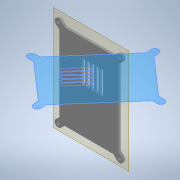
# Autodesk Inventor part: CoverWFan
Saved by Autodesk Inventor 2021 (Build 250183000, 183)
## iProperties
Created: 2021-07-24
Part Number: CoverWFan
Material: ABS Plastic
Document SubType Name: Modeling
Designer: cmzgt
Density: 1.06 g/cm^3
Appearance: Smooth - White
Author: cmzgt
Autodesk Inventor part; units mm, degrees
ref_plane "YZ Plane" through (0, 0, 0) normal (1, 0, 0) x (0, 1, 0)
ref_plane "XZ Plane" through (0, 0, 0) normal (0, 1, 0) x (-1, 0, 0)
ref_plane "XY Plane" through (0, 0, 0) normal (0, 0, 1) x (1, 0, 0)
ref_plane "Work Plane1" through (0, 0, 0) normal (0, 0, 1) x (1, 0, 0)
sketch "Sketch1" plane through (0, 0, 0) normal (0, 0, 1) x (1, 0, 0)
  line L0 (162.668, -44.5954) -> (162.668, 41.2818) projected
  line L1 (166.8059, 44.8966) -> (162.668, 41.2818) projected
  arc A0 (166.8059, 44.8966) -> (161.5426, 50.9214) centre (164.1742, 47.909) ccw projected
  circle A1 centre (164.1742, 47.909) radius 1.375 projected
  line L2 (158.5302, 48.2898) -> (161.5426, 50.9214) projected
  arc A2 (158.5302, 48.2898) -> (157.3844, 46.5932) centre (161.1618, 45.2774) ccw projected
  line L3 (157.3844, 46.5932) -> (101.3516, 46.5932) projected
  arc A3 (101.3516, 46.5932) -> (100.2059, 48.2898) centre (97.5742, 45.2774) ccw projected
  line L4 (97.1935, 50.9214) -> (100.2059, 48.2898) projected
  arc A4 (97.1935, 50.9214) -> (91.9302, 44.8966) centre (94.5618, 47.909) ccw projected
  circle A5 centre (94.5618, 47.909) radius 1.375 projected
  line L5 (96.068, 41.2818) -> (91.9302, 44.8966) projected
  line L6 (96.068, 41.2818) -> (96.068, -44.5954) projected
  line L7 (91.9302, -48.2102) -> (96.068, -44.5954) projected
  arc A6 (91.9302, -48.2102) -> (97.1935, -54.235) centre (94.5618, -51.2226) ccw projected
  line L8 (100.2059, -51.6034) -> (97.1935, -54.235) projected
  arc A7 (100.2059, -51.6034) -> (101.3516, -49.9068) centre (97.5742, -48.591) ccw projected
  circle A8 centre (94.5618, -51.2226) radius 1.375 projected
  line L9 (101.3516, -49.9068) -> (157.3844, -49.9068) projected
  line L10 (161.5426, -54.235) -> (158.5302, -51.6034) projected
  arc A9 (157.3844, -49.9068) -> (158.5302, -51.6034) centre (161.1618, -48.591) ccw projected
  arc A10 (161.5426, -54.235) -> (166.8059, -48.2102) centre (164.1742, -51.2226) ccw projected
  line L11 (162.668, -44.5954) -> (166.8059, -48.2102) projected
  circle A11 centre (164.1742, -51.2226) radius 1.375 projected
  line L12 (102.868, 42.7932) -> (155.868, 42.7932) projected
  arc A12 (158.868, 39.7932) -> (155.868, 42.7932) centre (155.868, 39.7932) ccw projected
  line L13 (158.868, 39.7932) -> (158.868, -43.1068) projected
  arc A13 (155.868, -46.1068) -> (158.868, -43.1068) centre (155.868, -43.1068) ccw projected
  line L14 (155.868, -46.1068) -> (102.868, -46.1068) projected
  arc A14 (99.868, -43.1068) -> (102.868, -46.1068) centre (102.868, -43.1068) ccw projected
  line L15 (99.868, -43.1068) -> (99.868, 39.7932) projected
  arc A15 (102.868, 42.7932) -> (99.868, 39.7932) centre (102.868, 39.7932) ccw projected
  point P0 (0, 0)
  point P1 (-32.2078, 42.9557)
  point P2 (-31.0209, 50.8588)
  point P3 (-31.2556, 42.9706)
  point P4 (90.7091, 46.8336)
  point P5 (90.8754, -49.6701)
  point P6 (94.8543, -45.6557)
  point P7 (38.6589, -48.4904)
  point P8 (35.6268, 48.0781)
extrude "Extrusion1" add sketch "Sketch1" along normal blind 2.5 contours L11 A10 L10 A9 L9 A7 L8 A6 L7 L6 L5 A4 L4 A3 L3 A2 L2 A0 L1 L0 | A1 | A5 | A8 | A11 | L12 A12 L13 A13 L14 A14 L15 A15
sketch "Sketch2" plane through (0, 0, 2.5) normal (0, 0, 1) x (1, 0, 0)
  line L0 (140.3574, 20.4135) -> (126.2672, 20.4135) construction
  line L1 (126.2672, 20.4135) -> (126.2672, 6.3233) construction
  line L2 (126.2672, 6.3233) -> (140.3574, 6.3233) construction
  line L3 (140.3574, 6.3233) -> (140.3574, 20.4135) construction
  line L4 (133.3123, 25.0032) -> (133.3123, 2.1432) construction
  line L5 (131.4073, 25.0032) -> (131.4073, 2.1432)
  line L6 (135.2173, 2.1432) -> (135.2173, 25.0032)
  arc A0 (135.2173, 25.0032) -> (131.4073, 25.0032) centre (133.3123, 25.0032) ccw
  arc A1 (131.4073, 2.1432) -> (135.2173, 2.1432) centre (133.3123, 2.1432) ccw
  line L7 (162.668, -44.5954) -> (162.668, 41.2818) projected
  line L8 (157.3844, 46.5932) -> (101.3516, 46.5932) projected
  line L9 (140.2973, 2.1432) -> (140.2973, 25.0032)
  arc A2 (140.2973, 25.0032) -> (136.4873, 25.0032) centre (138.3923, 25.0032) ccw
  line L10 (136.4873, 25.0032) -> (136.4873, 2.1432)
  arc A3 (136.4873, 2.1432) -> (140.2973, 2.1432) centre (138.3923, 2.1432) ccw
  line L11 (145.3773, 2.1432) -> (145.3773, 25.0032)
  arc A4 (145.3773, 25.0032) -> (141.5673, 25.0032) centre (143.4723, 25.0032) ccw
  line L12 (141.5673, 25.0032) -> (141.5673, 2.1432)
  arc A5 (141.5673, 2.1432) -> (145.3773, 2.1432) centre (143.4723, 2.1432) ccw
  arc A6 (130.1373, 25.0032) -> (126.3273, 25.0032) centre (128.2323, 25.0032) ccw
  line L13 (130.1373, 2.1432) -> (130.1373, 25.0032)
  line L14 (126.3273, 25.0032) -> (126.3273, 2.1432)
  arc A7 (126.3273, 2.1432) -> (130.1373, 2.1432) centre (128.2323, 2.1432) ccw
  arc A8 (125.0573, 25.0032) -> (121.2473, 25.0032) centre (123.1523, 25.0032) ccw
  line L15 (125.0573, 2.1432) -> (125.0573, 25.0032)
  line L16 (121.2473, 25.0032) -> (121.2473, 2.1432)
  arc A9 (121.2473, 2.1432) -> (125.0573, 2.1432) centre (123.1523, 2.1432) ccw
  circle A10 centre (94.5618, -51.2226) radius 1.375 projected
  circle A11 centre (164.1742, -51.2226) radius 1.375 projected
  circle A12 centre (164.1742, 47.909) radius 1.375 projected
  circle A13 centre (94.5618, 47.909) radius 1.375 projected
  point P0 (0, 0)
  point P1 (133.3123, 13.5732)
  dimension "d2" = 11.43
  dimension "d3" = 3.81
  dimension "d4" = 27.4507
  dimension "d5" = 21.59
  dimension "d6" = 14.0902
  dimension "d7" = 22.3106
  dimension "d8" = 36.4008
  dimension "d9" = 26.1797
  dimension "d12" = 5.08
  dimension "d19" = 5.08
  constraints: 32 end point, 20 point on circle, 10 centre point, 4 tangent, 3 horizontal, 3 parallel, 2 perpendicular, 1 midpoint, 40 other
  measures "d2" distance of point (133.312, 13.573) L4.end
  measures "d3" diameter of A1
  measures "d4" distance between parallel lines of L7 L6
  measures "d5" distance from line of L8 L4.start
  measures "d6" distance of L2.end L0.start
  measures "d7" distance between parallel lines of L3 L7
  measures "d8" distance between parallel lines of L1 L7
  measures "d9" distance between parallel lines of L0 L8
  measures "d12" distance of L6.start L9.start
  measures "d19" distance of L4.start A6.centre
extrude "Extrusion2" cut sketch "Sketch2" against normal up to surface (2.5 mm away)
body "Solid1"
